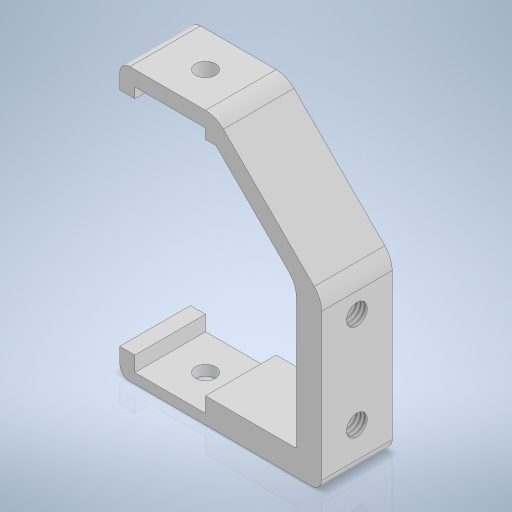
# Autodesk Inventor part: 114
Saved by Autodesk Inventor 2024 (Build 280153000, 153)
## iProperties
Created: 2024-06-07
Part Number: 114
Material: Generisch
Document SubType Name: Modeling
Designer: ffogue
Density: 1 g/cm^3
Appearance: Vorgabe
Author: ffogue
Autodesk Inventor part; units mm, degrees
ref_plane "YZ Plane" through (0, 0, 0) normal (1, 0, 0) x (0, 1, 0)
ref_plane "XZ Plane" through (0, 0, 0) normal (0, 1, 0) x (-1, 0, 0)
ref_plane "XY Plane" through (0, 0, 0) normal (0, 0, 1) x (1, 0, 0)
sketch "Skizze1" plane through (0, 0, 0) normal (0, 1, 0) x (-1, 0, 0)
  line L0 (0, -22) -> (0, -27)
  line L1 (0, -27) -> (-40, -27)
  line L2 (-40, -27) -> (-40, 4)
  line L3 (-17, 27) -> (0, 27)
  line L4 (0, 27) -> (0, 22)
  line L5 (0, -22) -> (-3, -22)
  line L6 (-3, -22) -> (-3, -25)
  line L7 (-3, -25) -> (-17, -25)
  line L8 (-17, -25) -> (-17, -22)
  line L9 (-17, -22) -> (-35, -22)
  line L10 (-35, -22) -> (-35, 4)
  line L11 (-17, 24) -> (-17, 24)
  line L12 (-17, 24) -> (-3, 24)
  line L13 (-3, 24) -> (-3, 22)
  line L14 (-3, 22) -> (0, 22)
  line L15 (0, 0) -> (-33.6444, 0) construction
  arc A0 (-33.5355, 7.5355) -> (-35, 4) centre (-30, 4) ccw
  line L16 (-33.5355, 7.5355) -> (-19.0711, 22)
  line L17 (-19.0711, 22) -> (-17, 22)
  line L18 (-17, 22) -> (-17, 24)
  line L19 (-17, 24) -> (-17, 24)
  arc A1 (-38.5355, 7.5355) -> (-40, 4) centre (-35, 4) ccw
  line L20 (-38.5355, 7.5355) -> (-20.5355, 25.5355)
  arc A2 (-17, 27) -> (-20.5355, 25.5355) centre (-17, 22) ccw
  point P0 (-1.5, 22)
  dimension "d2" = 5
  dimension "d3" = 40
  dimension "d4" = 3
  dimension "d5" = 14
  dimension "d6" = 54
  dimension "d7" = 3
  dimension "d8" = 2
  dimension "d12" = 26
  dimension "d16" = 2
  dimension "d17" = 3
  dimension "d18" = 5
  dimension "d19" = 5
  dimension "d20" = 5
  dimension "d21" = 45
  constraints: 43 end point, 11 perpendicular, 6 point on circle, 6 tangent, 5 vertical alignment, 4 point on line, 3 centre point, 2 horizontal, 2 horizontal alignment, 2 parallel, 2 vertical, 1 midpoint, 1 other
  measures "d2" distance between parallel lines of L2 L10
  measures "d3" distance between parallel lines of L2 L0
  measures "d4" distance of L0.start L5.end
  measures "d5" distance of L6.end L7.end
  measures "d6" distance between parallel lines of L1 L3
  measures "d7" distance between parallel lines of L7 L5
  measures "d8" distance between parallel lines of L1 L7
  measures "d12" distance of L9.end L10.end
  measures "d16" distance from line of point (-1.5, 22) L12
  measures "d17" distance between parallel lines of L3 L12
  measures "d18" radius of A0
  measures "d19" radius of A1
  measures "d20" radius of A2
  measures "d21" angle of L20 L2
extrude "Extrusion1" add sketch "Skizze1" along normal blind 14
fillet "Rundung1" radius 2 3 edges at (0, 7, -27) (40, 7, -27) (0, 7, 27)
fillet "Rundung2" radius 0.2 1 edges at (35, 7, -22)
sketch "Skizze2" plane through (35, 0, 4) normal (-1, 0, 0) x (0, 0, 1)
  line L0 (-31, 14) -> (-31, 0) projected
  point P0 (-4, 0)
  point P1 (-23, 7)
  point P2 (-4, 7)
  point P3 (-31, 7)
  dimension "d26" = 19
  dimension "d27" = 8
  constraints: 2 horizontal alignment, 1 midpoint
  measures "d26" distance of point (-23, 7) point (-4, 7)
  measures "d27" distance from line of L0 point (-23, 7)
hole "Bohrung1" at (35, 7, -19) at (35, 7, 0) direction (1, 0, 0) diameter 4.134 depth 5 thread size "M5x0.8" class "6H" standard "ISO Metric profile"
sketch "Skizze3" plane through (3, 0, -25) normal (0, 0, 1) x (1, 0, 0)
  line L0 (-3, 14) -> (-1, 14) projected
  line L1 (-1, 14) -> (-1, 0) projected
  line L2 (-1, 0) -> (-3, 0) projected
  line L3 (-3, 0) -> (-3, 14) projected
  point P0 (-3, 0)
  point P1 (7, 7)
  point P2 (-3, 7)
  dimension "d42" = 10
  constraints: 1 horizontal alignment, 1 midpoint
  measures "d42" distance from line of point (7, 7) L3
hole "Bohrung2" at (10, 7, -25) direction (0, 0, -1) diameter 4 end through all
sketch "Skizze5" plane through (17, 0, 24) normal (0, 0, -1) x (-1, 0, 0)
  line L0 (17, 14) -> (17, 0) projected
  point P0 (7, 7)
  point P1 (17, 7)
  dimension "d44" = 10
  constraints: 1 horizontal alignment, 1 midpoint
  measures "d44" distance from line of L0 point (7, 7)
hole "Bohrung3" at (10, 7, 24) direction (0, 0, 1) diameter 4 end through all
